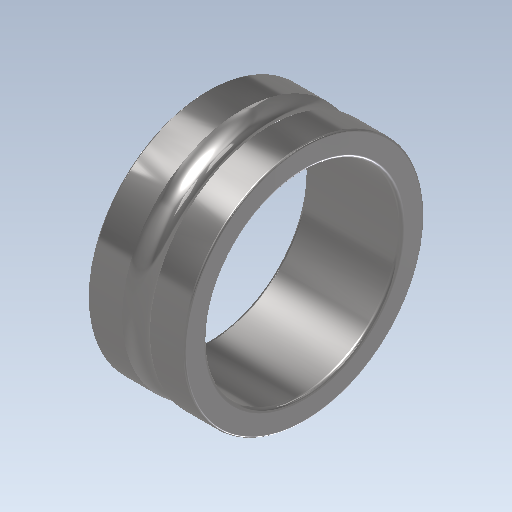
# Autodesk Inventor part: LF-1480ZZ_ir
Saved by Autodesk Inventor 2021 (Build 250183000, 183)
## iProperties
Created: 2019-07-28
Part Number: LF-1480ZZ_ir
Material: 鋼、炭素鋼
Catalog Web Link: www.cadenas.de
Description: Radial Flanged Ball Bearings (RF-Series/LF series) Metric ST ir-Radial Flanged Ball Bearings (RF-Series/LF series) Metric Shielded Type
Vendor: NMB
Document SubType Name: Modeling
Designer: psadmin
Manufacturer: NMB
Mass: 0.790149 g
Surface Area: 2.76007 cm^2
Volume: 0.100656 cm^3
Density: 7.85 g/cm^3
Appearance: 半つや出し
Category: PARTsolutions
Company: NMB
PSOL_IDENT_0: {$CADENAS_DATA\23d-libs\nmb\pbbp\radial_flanged_ball_bearings\rfbb_rflfs_m\rflf_shielded_ir.prj},223
PSOL_IDENT_1: {VTYP=3D},{NB=LF-1480ZZ_ir},{LINA=LF-1480ZZ_ir},{NN=Radial Flanged Ball Bearings (RF-Series/LF seri
PSOL_IDENT_2: es) Metric ST ir},{DATE=11.11.2013 05:13:45},{GEOMDATE=24.10.2013 10:33:00},{VERSION=},{LINEID=1270}
PSOL_IDENT_3: ,{WBVAR=},{WBNUMERIC=}  {NB=LF-1480ZZ_ir},{LINA=LF-1480ZZ_ir},{KT=DUMMY},{IDNR=},{PN=LF-1480ZZ},{SHL
PSOL_IDENT_4: D=shielded},{FLANG=flanged},{SD=8.000},{D=14.000},{B=4.000},{SR=0.15},{BCZ=10},{DW=1.5875},{LI=9.90}
PSOL_IDENT_5: ,{LO=12.55},{D1=15.600},{C1=0.80},{D2=0.0},{C2=0.00},{COR=386},{CR=1036},{PCD=11.000},{U=12.588},{W=
PSOL_IDENT_6: 9.413},{Y=0.794},{Z=0.794},{AA=12.429},{AC=0.80},{AD=0.000},{AF=0.00},{AQ=0.20},{AH=12.75},{AI=10.10
PSOL_IDENT_7: },{AJ=0.40}
NN: Radial Flanged Ball Bearings (RF-Series/LF series) Metric ST ir
NT: Radial Flanged Ball Bearings (RF-Series/LF series) Metric Shielded Type
NB: LF-1480ZZ_ir
NBSYN: $PN._ir
LINA: LF-1480ZZ_ir
PN: LF-1480ZZ
SHLD: shielded
FLANG: flanged
SD: 8
D: 14
B: 4
SR: 0.15
BCZ: 10
DW: 1.5875
LI: 9.9
LO: 12.55
D1: 0
C1: 0.8
D2: 0
C2: 0
COR: 386
CR: 1036
PCD: 11
U: 12.588
W: 9.413
Y: 0.794
Z: 0.794
AA: 12.429
AC: 0.8
AD: 0
AF: 0
AQ: 0.2
AH: 12.75
AI: 10.1
AJ: 0.4
SUPPLIER: NMB
ARTICLENO: LF-1480ZZ_ir
BOMINFO: LF-1480ZZ_ir
CREATOR: CADENAS GmbH
Title: LF-1480ZZ_ir
Author: Cadenas PARTsolutions
Comments: Radial Flanged Ball Bearings (RF-Series/LF series) Metric Shielded Type
Autodesk Inventor part; units mm, degrees
sketch "Sketch_5" plane through (0, 0, 0) normal (0, 0, 1) x (1, 0, 0)
  line L0 (4, 0) -> (0, 0)
  line L1 (0, 4.875) -> (0, 4.15)
  arc A0 (0, 4.15) -> (0.15, 4) centre (0.15, 4.15) ccw
  line L2 (0.15, 4) -> (3.85, 4)
  arc A1 (3.85, 4) -> (4, 4.15) centre (3.85, 4.15) ccw
  line L3 (4, 4.15) -> (4, 4.875)
  arc A2 (4, 4.875) -> (3.925, 4.95) centre (3.925, 4.875) ccw
  line L4 (3.925, 4.95) -> (2.5723, 4.95)
  arc A3 (1.4277, 4.95) -> (2.5723, 4.95) centre (2, 5.5) ccw
  line L5 (1.4277, 4.95) -> (0.075, 4.95)
  arc A4 (0.075, 4.95) -> (0, 4.875) centre (0.075, 4.875) ccw
  constraints: 12 end point, 10 point on circle, 5 centre point
revolve "Revolution1" add sketch "Sketch_5" angle 360 about axis through (4, 0, 0) along (1, 0, 0)
ref_plane "1_XY" through (2, 0, 0) normal (1, 0, 0) x (0, 0, -1)
ref_plane "1_YZ" through (2, 0, 0) normal (0, 0, -1) x (0, 1, 0)
ref_plane "1_ZX" through (2, 0, 0) normal (0, 1, 0) x (1, 0, 0)
ref_plane "Dummy_XY" through (0, 0, 0) normal (1, 0, 0) x (0, 0, -1)
ref_plane "Dummy_YZ" through (0, 0, 0) normal (0, 0, -1) x (0, 1, 0)
ref_plane "Dummy_ZX" through (0, 0, 0) normal (0, 1, 0) x (1, 0, 0)
ref_plane "shield1_XY" through (0.4, 0, 0) normal (1, 0, 0) x (0, 0, -1)
ref_plane "shield1_YZ" through (0.4, 0, 0) normal (0, 0, -1) x (0, 1, 0)
ref_plane "shield1_ZX" through (0.4, 0, 0) normal (0, 1, 0) x (1, 0, 0)
ref_plane "shield2_XY" through (3.6, 0, 0) normal (-1, 0, 0) x (0, 0, -1)
ref_plane "shield2_YZ" through (3.6, 0, 0) normal (0, 0, -1) x (0, -1, 0)
ref_plane "shield2_ZX" through (3.6, 0, 0) normal (0, -1, 0) x (-1, 0, 0)
body "Solid1"
